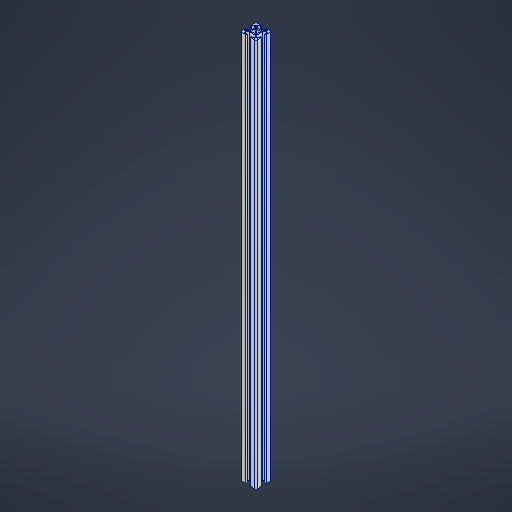
# Autodesk Inventor part: SIDE_BEAMSipt-01
Saved by Autodesk Inventor 2026.2 (Build 302298010, 298A)
## iProperties
Created: 2026-02-11
Part Number: SIDE_BEAMSipt-01
Material: Aluminum 6061
Document SubType Name: Modeling
Designer: Luke
Density: 2.7 g/cm^3
Appearance: Aluminum - Flat
Author: Luke
Autodesk Inventor part; units mm, degrees
ref_plane "YZ Plane" through (0, 0, 0) normal (1, 0, 0) x (0, 1, 0)
ref_plane "XZ Plane" through (0, 0, 0) normal (0, 1, 0) x (-1, 0, 0)
ref_plane "XY Plane" through (0, 0, 0) normal (0, 0, 1) x (1, 0, 0)
sketch "Sketch1" plane through (0, 0, 0) normal (0, 1, 0) x (-1, 0, 0)
  line L0 (-8.5066, -10.0066) -> (8.5066, -10.0066)
  line L1 (10.0066, -9.9934) -> (10.0066, 8.5066) construction
  line L2 (8.5066, 10.0066) -> (-9.9934, 10.0066) construction
  line L3 (-10.0066, 8.5066) -> (-10.0066, -8.5066)
  line L4 (-10.0066, -10.0066) -> (10.0066, 10.0066) construction
  line L5 (10.0066, -9.9934) -> (-9.5735, 9.5609) construction
  line L6 (-3.5, -4.5607) -> (3.5, -4.5607)
  line L7 (4.5607, -3.5) -> (4.5607, 3.5)
  line L8 (3.5, 4.5607) -> (-3.5, 4.5607)
  line L9 (-4.5607, 3.5) -> (-4.5607, -3.5)
  line L10 (-4.75, -4.75) -> (4.75, 4.75) construction
  line L11 (8.5066, 10.0066) -> (6.1559, 10.0066)
  line L12 (5.9459, 8.5066) -> (5.9459, 7.0066)
  line L13 (7.0066, 5.9459) -> (8.5066, 5.9459)
  line L14 (10.0066, 6.164) -> (10.0066, 8.5066)
  line L15 (-3.25, -3.25) -> (3.25, 3.25) construction
  line L16 (3.25, -3.25) -> (-3.25, 3.25) construction
  line L17 (0, 0) -> (20.0131, 20.0131) construction
  line L18 (8.5066, 5.9459) -> (8.5066, 3.0066)
  line L19 (8.5066, 3.0066) -> (10.0066, 3.0066)
  line L20 (10.0066, 3.0066) -> (10.0066, 6.164)
  line L21 (6.1559, 10.0066) -> (3.0066, 10.0066)
  line L22 (3.0066, 10.0066) -> (3.0066, 8.5066)
  line L23 (3.0066, 8.5066) -> (5.9459, 8.5066)
  arc A0 (10.0066, 8.5066) -> (8.5066, 10.0066) centre (8.5066, 8.5066) ccw
  line L24 (0, -13.1094) -> (0, 17.292) construction
  line L25 (14.9507, 0) -> (-14.3529, 0) construction
  circle A1 centre (0, 0) radius 4.5962 construction
  line L26 (4.5607, 3.5) -> (7.0066, 5.9459)
  line L27 (3.5, 4.5607) -> (5.9459, 7.0066)
  line L28 (5.7658, 4.7051) -> (5.2355, 5.2355) construction
  line L29 (3.0066, 10.0066) -> (8.5066, 10.0066)
  line L30 (10.0066, 3.0066) -> (10.0066, 8.5066)
  line L31 (-88.3377, -18.3534) -> (-20.6276, -18.3534) construction
  line L32 (-20.6276, -18.3534) -> (-20.6276, -138.727) construction
  line L33 (-20.6276, -138.727) -> (-88.3377, -138.727) construction
  line L34 (-88.3377, -138.727) -> (-88.3377, -18.3534) construction
  line L35 (-10.0066, 8.5066) -> (-10.0066, 6.1559)
  arc A2 (-8.5066, 10.0066) -> (-10.0066, 8.5066) centre (-8.5066, 8.5066) ccw
  line L36 (-6.164, 10.0066) -> (-8.5066, 10.0066)
  line L37 (9.9934, 10.0066) -> (-8.5066, 10.0066) construction
  line L38 (-3.0066, 10.0066) -> (-6.164, 10.0066)
  line L39 (-5.9459, 8.5066) -> (-3.0066, 8.5066)
  line L40 (-3.0066, 8.5066) -> (-3.0066, 10.0066)
  line L41 (-5.9459, 7.0066) -> (-5.9459, 8.5066)
  line L42 (-3.5, 4.5607) -> (-5.9459, 7.0066)
  line L43 (-4.5607, 3.5) -> (-7.0066, 5.9459)
  line L44 (-8.5066, 5.9459) -> (-7.0066, 5.9459)
  line L45 (-8.5066, 3.0066) -> (-8.5066, 5.9459)
  line L46 (-10.0066, 8.5066) -> (-10.0066, -9.9934) construction
  line L47 (-10.0066, 3.0066) -> (-8.5066, 3.0066)
  line L48 (-10.0066, 6.1559) -> (-10.0066, 3.0066)
  line L49 (-8.5066, -10.0066) -> (-6.1559, -10.0066)
  arc A3 (-10.0066, -8.5066) -> (-8.5066, -10.0066) centre (-8.5066, -8.5066) ccw
  line L50 (-10.0066, -6.164) -> (-10.0066, -8.5066)
  line L51 (-10.0066, 9.9934) -> (-10.0066, -8.5066) construction
  line L52 (-10.0066, -3.0066) -> (-10.0066, -6.164)
  line L53 (-8.5066, -5.9459) -> (-8.5066, -3.0066)
  line L54 (-8.5066, -3.0066) -> (-10.0066, -3.0066)
  line L55 (-7.0066, -5.9459) -> (-8.5066, -5.9459)
  line L56 (-4.5607, -3.5) -> (-7.0066, -5.9459)
  line L57 (-3.5, -4.5607) -> (-5.9459, -7.0066)
  line L58 (-5.9459, -8.5066) -> (-5.9459, -7.0066)
  line L59 (-3.0066, -8.5066) -> (-5.9459, -8.5066)
  line L60 (-8.5066, -10.0066) -> (9.9934, -10.0066) construction
  line L61 (-3.0066, -10.0066) -> (-3.0066, -8.5066)
  line L62 (-6.1559, -10.0066) -> (-3.0066, -10.0066)
  line L63 (10.0066, -8.5066) -> (10.0066, -6.1559)
  arc A4 (8.5066, -10.0066) -> (10.0066, -8.5066) centre (8.5066, -8.5066) ccw
  line L64 (6.164, -10.0066) -> (8.5066, -10.0066)
  line L65 (-9.9934, -10.0066) -> (8.5066, -10.0066) construction
  line L66 (3.0066, -10.0066) -> (6.164, -10.0066)
  line L67 (5.9459, -8.5066) -> (3.0066, -8.5066)
  line L68 (3.0066, -8.5066) -> (3.0066, -10.0066)
  line L69 (5.9459, -7.0066) -> (5.9459, -8.5066)
  line L70 (3.5, -4.5607) -> (5.9459, -7.0066)
  line L71 (4.5607, -3.5) -> (7.0066, -5.9459)
  line L72 (8.5066, -5.9459) -> (7.0066, -5.9459)
  line L73 (8.5066, -3.0066) -> (8.5066, -5.9459)
  line L74 (10.0066, -8.5066) -> (10.0066, 9.9934) construction
  line L75 (10.0066, -3.0066) -> (8.5066, -3.0066)
  line L76 (10.0066, -6.1559) -> (10.0066, -3.0066)
  line L77 (-3.6951, -3.0204) -> (-3.0204, -3.6951)
  line L78 (-3.0204, -3.6951) -> (3.0204, 3.6951) construction
  line L79 (3.6951, 3.0204) -> (-3.6951, -3.0204) construction
  line L80 (3.7133, -3.0016) -> (3.0065, -3.7094)
  line L81 (3.0065, -3.7094) -> (-3.1656, 3.9057) construction
  line L82 (-3.8767, 3.1337) -> (3.7133, -3.0016) construction
  line L83 (3.7133, -3.0016) -> (3.0065, -3.7094)
  line L84 (0.4404, 0.4404) -> (0.8591, 0)
  line L85 (3.25, -2.5143) -> (3.7133, -3.0016)
  line L86 (3.0065, -3.7094) -> (2.5696, -3.25)
  line L87 (0, -0.5477) -> (-0.267, -0.267)
  line L88 (3.25, -3.25) -> (3.25, -3.2457)
  line L89 (3.25, -2.5143) -> (3.25, 2.5696)
  line L90 (2.5143, 3.25) -> (3.0016, 3.7133)
  line L91 (3.0016, 3.7133) -> (3.7094, 3.0065)
  line L92 (3.7094, 3.0065) -> (3.25, 2.5696)
  line L93 (-3.25, 2.5143) -> (-3.7133, 3.0016)
  line L94 (-3.7133, 3.0016) -> (-3.0065, 3.7094)
  line L95 (-3.0065, 3.7094) -> (-2.5696, 3.25)
  line L96 (-2.5143, -3.25) -> (-3.0016, -3.7133)
  line L97 (-3.0016, -3.7133) -> (-3.7094, -3.0065)
  line L98 (-3.7094, -3.0065) -> (-3.25, -2.5696)
  line L99 (-2.5143, -3.25) -> (2.5696, -3.25)
  line L100 (-3.25, 3.25) -> (-3.25, 3.2457)
  line L101 (-3.25, 2.5143) -> (-3.25, -2.5696)
  line L102 (2.5143, 3.25) -> (-2.5696, 3.25)
  point P0 (5.9459, 7.7566)
  point P1 (-10.0066, 10.0066)
  point P2 (-4.7051, 5.7658)
  point P3 (-7.7566, 5.9459)
  point P4 (-10.0066, -10.0066)
  point P5 (-5.7658, -4.7051)
  point P6 (-5.9459, -7.7566)
  point P7 (10.0066, -10.0066)
  point P8 (4.7051, -5.7658)
  point P9 (7.7566, -5.9459)
  point P10 (3.3599, -3.3555)
  point P11 (0.5158, 0.631)
  point P12 (3.3555, 3.3599)
  point P13 (-3.3599, 3.3555)
  point P14 (-3.3555, -3.3599)
  dimension "d0" = 20
  dimension "d1" = 1.5
  dimension "d2" = 1.5
  dimension "d3" = 1.5
  dimension "d4" = 0.75
  dimension "d5" = 7
  dimension "d6" = 7
  dimension "d46" = 1.5
  dimension "d57" = 360
  dimension "d61" = 7
  dimension "d66" = 360
  constraints: 198 end point, 26 point on line, 19 parallel, 10 midpoint, 10 perpendicular, 9 point on circle, 6 horizontal, 4 centre point, 4 equal length, 2 collinear, 2 tangent, 1 coincident, 1 vertical, 179 other
  measures "d0" distance of L4.end L2.end
  measures "d1" distance between parallel lines of L18 L20
  measures "d2" radius of A0
  measures "d3" distance between parallel lines of L27 L26
  measures "d4" distance between parallel lines of L17 L27
  measures "d5" distance of L21.end point (10.007, 10.007)
  measures "d6" distance of L19.end L4.end
  measures "d46" distance of L12.start L12.end
  measures "d61" distance of L8.start L8.end
extrude "Extrusion1" add sketch "Sketch1" along normal blind 500 contours A3 L3 L54 L53 L55 L56 L9 L43 L44 L45 L47 A2 L36 L38 L40 L39 L41 L42 L8 L27 L12 L23 L22 L21 L11 A0 L14 L20 L19 L18 L13 L26 L7 L71 L72 L73 L75 L76 L63 A4 L0 L68 L67 L69 L70 L6 L57 L58 L59 L61
body "Solid1"
